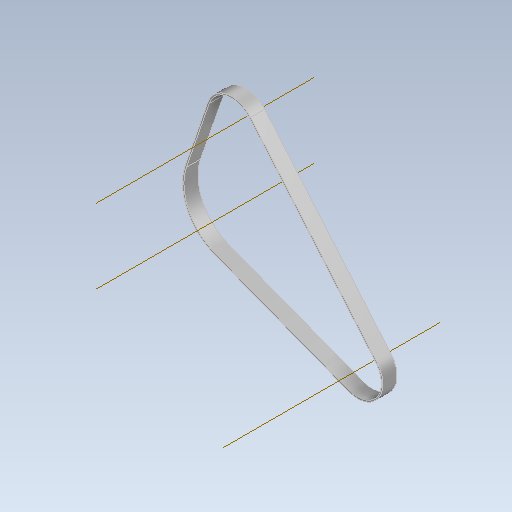
# Autodesk Inventor part: Зубчатый ремень
Saved by Autodesk Inventor 2021 (Build 250183000, 183)
## iProperties
Created: 2021-06-15
Part Number: Зубчатый ремень
Material: Rubber
Document SubType Name: Modeling
Designer: panda
Density: 1 g/cm^3
Appearance: Rubber - Black - Version 1.1
CustomPartVersion: 1
Author: panda
Autodesk Inventor part; units mm, degrees
sketch "Эскизная траектория" plane through (0, 0, 0) normal (0, 0, 1) x (1, 0, 0)
  arc A0 (41.6799, 153.6758) -> (-13.5638, 143.1896) centre (17.0385, 132.7307) ccw
  arc A1 (175.434, -97.4559) -> (211.6799, -46.3242) centre (187.0385, -67.2693) ccw
  arc A2 (-44.1662, 53.6486) -> (-6.1705, -27.6425) centre (17.0385, 32.7307) ccw
  line L0 (-44.1662, 53.6486) -> (-13.5638, 143.1896)
  line L1 (41.6799, 153.6758) -> (211.6799, -46.3242)
  line L2 (175.434, -97.4559) -> (-6.1705, -27.6425)
  constraints: 6 end point, 6 point on circle, 3 centre point
ref_plane "Плоскость сечения" through (-13.5638, 143.1896, 0) normal (-0.3234, -0.9463, 0) x (0, 0, 1)
ref_plane "РабПлоскость2" through (17.0385, 132.7307, 0) normal (-1, 0, 0) x (0, 0, 1)
ref_plane "РабПлоскость3" through (187.0385, -67.2693, 0) normal (-0.6093, 0.7929, 0) x (0, 0, 1)
ref_plane "РабПлоскость4" through (17.0385, 32.7307, 0) normal (0.9279, -0.3729, 0) x (0, 0, 1)
sketch "Сечение" plane through (-13.5638, 143.1896, 0) normal (-0.3234, -0.9463, 0) x (0, 0, 1)
  line L0 (-9.525, 1.3462) -> (9.525, 1.3462)
  line L1 (9.525, 1.3462) -> (9.525, -0.6858)
  line L2 (9.525, -0.6858) -> (-9.525, -0.6858)
  line L3 (-9.525, -0.6858) -> (-9.525, 1.3462)
  line L4 (-9.525, 0) -> (9.525, 0) construction
  point P0 (0, 0)
  point P1 (0, 0)
  dimension "d0" = 19.05
  dimension "d4" = 0.6858
  dimension "d5" = 1.3462
  constraints: 10 end point, 2 parallel, 2 point on line, 1 coincident, 1 horizontal, 1 midpoint, 1 perpendicular, 1 other
  measures "d0" distance between parallel lines of L1 L3
  measures "d4" distance between parallel lines of L2 L4
  measures "d5" distance between parallel lines of L4 L0
sweep "Ремень" add profiles "Сечение" path "Эскизная траектория"
equation "\"d0\" = da_B"
equation "\"d4\" = da_a"
equation "\"d5\" = da_a2"
equation "\"da_B\" = 19.05"
equation "\"da_pb\" = 12.7"
equation "\"da_L\" = 804.4568"
equation "\"da_a\" = 0.6858"
equation "\"da_S\" = 6.1214"
equation "\"da_Beta\" = 20deg"
equation "\"da_Ht\" = 2.286"
equation "\"da_H\" = 4.318"
equation "\"da_a2\" = 1.3462"
body "Solid1"
